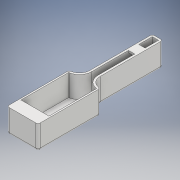
# Autodesk Inventor part: POVwand
Saved by Autodesk Inventor 2017 SP1 (Build 210196100, 196)
## iProperties
Created: 2016-11-21
Part Number: POVwand
Material: ABS Plastic
Document SubType Name: Modeling
Designer: bzs3334
Density: 1.06 g/cm^3
Appearance: Smooth - White
Mass: 17.3028 g
Surface Area: 186.157 cm^2
Volume: 16.3234 cm^3
Author: bzs3334
Autodesk Inventor part; units mm, degrees
ref_plane "YZ Plane" through (0, 0, 0) normal (1, 0, 0) x (0, 1, 0)
ref_plane "XZ Plane" through (0, 0, 0) normal (0, 1, 0) x (-1, 0, 0)
ref_plane "XY Plane" through (0, 0, 0) normal (0, 0, 1) x (1, 0, 0)
sketch "Sketch1" plane through (0, 0, 0) normal (0, 0, 1) x (1, 0, 0)
  line L0 (-5, 0) -> (5, 0)
  line L1 (5, 10) -> (5, 115)
  line L2 (5, 115) -> (-5, 115)
  line L3 (-5, 115) -> (-5, 10)
  line L4 (-15, 0) -> (15, 0)
  line L5 (15, 0) -> (15, -60)
  line L6 (15, -60) -> (-15, -60)
  line L7 (-15, -60) -> (-15, 0)
  arc A0 (-15, 0) -> (-5, 10) centre (-15, 10) ccw
  line L8 (-15, 0) -> (-5, 10) construction
  line L9 (-15, 0) -> (-0.8579, 0) construction
  line L10 (0, 0) -> (0, 115)
  arc A1 (5, 10) -> (15, 0) centre (15, 10) ccw
  circle A2 centre (0, 65) radius 2.7
  circle A3 centre (0, 58.6) radius 2.7
  circle A4 centre (0, 52.2) radius 2.7
  circle A5 centre (0, 45.8) radius 2.7
  circle A6 centre (0, 39.4) radius 2.7
  circle A7 centre (0, 33) radius 2.7
  circle A8 centre (0, 26.6) radius 2.7
  circle A9 centre (0, 20.2) radius 2.7
  circle A10 centre (0, 13.8) radius 2.7
  circle A11 centre (0, 7.4) radius 2.7
  circle A12 centre (0, 1) radius 2.7
  line L11 (5, 68.5) -> (-5, 68.5)
  dimension "a" = 10
  dimension "d1" = 115
  dimension "d2" = 5
  dimension "d3" = 60
  dimension "b" = 30
  dimension "d6" = 15
  dimension "d7" = 45
  dimension "d10" = 5.4
  dimension "d11" = 50
  dimension "d14" = 6.4
  dimension "d47" = 3.5
  constraints: 24 end point, 13 centre point, 4 parallel, 4 point on circle, 4 point on line, 3 horizontal, 3 perpendicular, 2 symmetric about line, 2 tangent, 1 equal length, 1 midpoint, 1 vertical, 21 other
  measures "a" distance between parallel lines of L3 L1
  measures "d1" distance of L0.end L1.end
  measures "d2" distance from line of L10.start L1
  measures "d3" distance of L4.end L5.end
  measures "b" distance of L5.end L6.end
  measures "d6" distance from line of L10.start L5
  measures "d7" angle of L9 L8
  measures "d10" diameter of A2
  measures "d11" distance of L10.end A2.centre
  measures "d14" distance of A2.centre A3.centre
  measures "d47" distance from line of L11 A2.centre
extrude "Extrusion1" add sketch "Sketch1" along normal blind 23
sketch "Sketch2" plane through (0, 0, 23) normal (0, 0, 1) x (1, 0, 0)
  line L0 (5, 115) -> (-5, 115) projected
  line L1 (-5, 115) -> (-5, 10) projected
  arc A0 (-15, 0) -> (-5, 10) centre (-15, 10) ccw projected
  line L2 (-15, 0) -> (-15, -60) projected
  line L3 (-15, -60) -> (15, -60) projected
  line L4 (15, -60) -> (15, 0) projected
  arc A1 (5, 10) -> (15, 0) centre (15, 10) ccw projected
  line L5 (5, 10) -> (5, 115) projected
  line L6 (-13, -28) -> (-13, -1.8322)
  arc A2 (-13, -1.8322) -> (-3, 10) centre (-15, 10) ccw
  line L7 (-3, 10) -> (-3, 113)
  line L8 (-3, 113) -> (3, 113)
  line L9 (3, 113) -> (3, 10)
  arc A3 (3, 10) -> (13, -1.8322) centre (15, 10) ccw
  line L10 (13, -1.8322) -> (13, -28)
  line L11 (-15, 0) -> (-15, -60) projected
  line L12 (-15, -28) -> (13, -28)
  point P0 (0, 0)
  dimension "d19" = 2
  constraints: 12 end point, 4 point on circle, 2 centre point, 1 point on line, 4 other
  measures "d19" distance between parallel lines of L2 L6
extrude "Extrusion2" cut sketch "Sketch2" against normal blind 21 contours L6 A2 L7 L8 L9 A3 L10 L12
sketch "Sketch3" plane through (-13, -28, 23) normal (0, 1, 0) x (1, 0, 0)
  line L0 (-2, 23) -> (28, 23) projected
  line L1 (28, 23) -> (28, 0) projected
  line L2 (-2, 0) -> (28, 0) projected
  line L3 (-2, 23) -> (-2, 0) projected
  line L4 (26, 2) -> (26, 21)
  line L5 (26, 21) -> (0, 21)
  line L6 (0, 21) -> (0, 2)
  line L7 (0, 2) -> (26, 2)
  point P0 (13, 23)
  dimension "d23" = 2
  constraints: 8 end point, 3 other
  measures "d23" distance between parallel lines of L2 L7
extrude "Extrusion3" cut sketch "Sketch3" against normal blind 30 contours L7 L6 L5 L4
extrude "Extrusion4" cut sketch "Sketch1" along normal through all contours A12 L10 L0 | L0 A12 | L10 A12 L0 | A11 L10 | L10 A11 | A10 L10 | L10 A10 | A2 L10 | L10 A2 | A9 L10 | L10 A9 | A3 L10 | L10 A3 | A8 L10 | L10 A8 | A4 L10 | L10 A4 | A7 L10 | L10 A7 | A5 L10 | L10 A5 | A6 L10 | L10 A6
fillet "Fillet1" radius 2 1 edges at (15, 0, 11.5)
mirror "Mirror1" about plane through (0, 0, 0) normal (1, 0, 0) of "Fillet1"
fillet "Fillet2" radius 2 2 edges at (-15, -60, 11.5) (15, -60, 11.5)
fillet "Fillet4" radius 2 2 edges at (5, 115, 11.5) (-5, 115, 11.5)
fillet "Fillet5" radius 2 14 edges at (-7.3624, 3.545, 0) (-14.5275, -0.5412, 0) (-15, -29.9161, 0) (-14.4142, -59.4142, 0) (0, -60, 0) (14.4142, -59.4142, 0) (15, -29.9161, 0) (14.5275, -0.5412, 0) (7.3624, 3.545, 0) (5, 61.5, 0) (4.4142, 114.4142, 0) (0, 115, 0) (-4.4142, 114.4142, 0) (-5, 61.5, 0)
sketch "Sketch4" plane through (-13, -28, 23) normal (1, 0, 0) x (0, 0, -1)
  line L0 (21, -30) -> (21, 26.1678) projected
  line L1 (0, -30) -> (21, -30) projected
  line L2 (0, 26.1678) -> (0, -30) projected
  line L3 (21, 26.1678) -> (0, 26.1678) projected
  point P0 (23, 28)
sketch "Sketch5" plane through (-13, -28, 23) normal (1, 0, 0) x (0, 0, -1)
  line L0 (0, 0) -> (2, 0) projected
  line L1 (2, 0) -> (2, -30) projected
  point P0 (23, 28)
sketch "Sketch6" plane through (-13, -28, 23) normal (0, 1, 0) x (1, 0, 0)
  line L0 (26, 2) -> (0, 2) projected
  line L1 (0, 0) -> (26, 0) projected
  line L2 (26, 0) -> (26, 21) projected
  line L3 (0, 0) -> (26, 0)
  line L4 (26, 0) -> (26, 2)
  line L5 (26, 2) -> (0, 2)
  line L6 (0, 2) -> (0, 0)
  point P0 (13, 23)
  constraints: 8 end point, 2 parallel, 1 horizontal, 1 perpendicular
extrude "Extrusion5" cut sketch "Sketch6" against normal blind 10
extrude "Extrusion6" cut sketch "Sketch4" against normal blind 0.5
mirror "Mirror2" about plane through (0, 0, 0) normal (1, 0, 0) of "Extrusion6"
sketch "Sketch9" plane through (13, -58, 23) normal (1, 0, 0) x (0, 0, -1)
  line L0 (2, 20) -> (2, 0) projected
  line L1 (2, 0) -> (0, 0) projected
  line L2 (0, 20) -> (0, 0) projected
  line L3 (0, 20) -> (2, 20) projected
  point P0 (23, 58)
extrude "Extrusion7" add sketch "Sketch9" along normal blind 0.5
mirror "Mirror3" about plane through (0, 0, 0) normal (1, 0, 0) of "Extrusion7"
sketch "Sketch10" plane through (0, 0, 23) normal (0, 0, 1) x (1, 0, 0)
  arc A0 (-3, 115) -> (-5, 113) centre (-3, 113) ccw projected
  line L0 (-5, 113) -> (-5, 10) projected
  arc A1 (-13.3333, 0.1399) -> (-5, 10) centre (-15, 10) ccw projected
  arc A2 (-13.3333, 0.1399) -> (-15, -1.8322) centre (-13, -1.8322) ccw projected
  line L1 (-15, -1.8322) -> (-15, -58) projected
  arc A3 (-15, -58) -> (-13, -60) centre (-13, -58) ccw projected
  line L2 (-13, -60) -> (13, -60) projected
  arc A4 (13, -60) -> (15, -58) centre (13, -58) ccw projected
  line L3 (15, -58) -> (15, -1.8322) projected
  arc A5 (15, -1.8322) -> (13.3333, 0.1399) centre (13, -1.8322) ccw projected
  arc A6 (5, 10) -> (13.3333, 0.1399) centre (15, 10) ccw projected
  line L4 (5, 10) -> (5, 113) projected
  arc A7 (5, 113) -> (3, 115) centre (3, 113) ccw projected
  line L5 (3, 115) -> (-3, 115) projected
  line L6 (13, -1.8322) -> (13.5, -1.8322) projected
  line L7 (13.5, -1.8322) -> (13.5, -38) projected
  line L8 (13.5, -38) -> (-13.5, -38) projected
  line L9 (-13.5, -38) -> (-13.5, -1.8322) projected
  line L10 (-13.5, -1.8322) -> (-13, -1.8322) projected
  arc A8 (-13, -1.8322) -> (-3, 10) centre (-15, 10) ccw projected
  line L11 (-3, 10) -> (-3, 113) projected
  line L12 (-3, 113) -> (3, 113) projected
  line L13 (3, 113) -> (3, 10) projected
  arc A9 (3, 10) -> (13, -1.8322) centre (15, 10) ccw projected
  line L14 (-13.5, -38) -> (-13.5, -1.8322) projected
  line L15 (13.5, -58) -> (13.5, -38) projected
  line L16 (-13.5, -38) -> (13.5, -38)
  line L17 (13.5, -38) -> (13.5, -48)
  line L18 (13.5, -48) -> (-13.5, -48)
  line L19 (-13.5, -48) -> (-13.5, -38)
  point P0 (0, 0)
  dimension "d53" = 10
  constraints: 8 end point, 2 parallel, 1 horizontal, 1 midpoint, 1 perpendicular
  measures "d53" distance of L16.end L17.end
sketch "Sketch11" plane through (-13, -38, 23) normal (0, 1, 0) x (1, 0, 0)
  line L0 (-0.5, 2) -> (26.5, 2) projected
  line L1 (26, 21) -> (0, 21) projected
  line L2 (26, 0) -> (26, 21) projected
  line L3 (0, 0) -> (26, 0) projected
  line L4 (0, 21) -> (0, 0) projected
  line L5 (0, 21) -> (0, 0) projected
  line L6 (26, 0) -> (26, 21) projected
  line L7 (0, 2) -> (26, 2)
  line L8 (26, 2) -> (26, 1.5)
  line L9 (26, 1.5) -> (0, 1.5)
  line L10 (0, 1.5) -> (0, 2)
  line L11 (-0.5, 21) -> (-0.5, 2) projected
  line L12 (0, 1.5) -> (-0.5, 1.5)
  line L13 (-0.5, 1.5) -> (-0.5, 2)
  line L14 (-0.5, 2) -> (0, 2)
  line L15 (0, 2) -> (0, 1.5)
  point P0 (13, 23)
  dimension "d39" = 0.5
  constraints: 16 end point, 4 parallel, 3 point on line, 2 horizontal, 2 perpendicular
  measures "d39" distance of L7.end L8.end
extrude "Extrusion8" cut sketch "Sketch11" against normal blind 20 contours L0 L4 L12 L13 | L0 L2 L9 L4
sketch "Sketch12" plane through (-3, 10, 23) normal (1, 0, 0) x (0, 0, -1)
  line L0 (21, 0) -> (21, 103) projected
  line L1 (21, 0) -> (0, 0) projected
  line L2 (0, 103) -> (0, 0) projected
  line L3 (21, 103) -> (0, 103) projected
  line L4 (0, 103) -> (0, 0) projected
  line L5 (0, 35.5) -> (2, 35.5)
  line L6 (2, 35.5) -> (2, 45.5)
  line L7 (2, 45.5) -> (0, 45.5)
  line L8 (0, 45.5) -> (0, 35.5)
  point P0 (23, -10)
  dimension "d42" = 2
  dimension "d43" = 10
  dimension "d44" = 57.5
  constraints: 8 end point, 2 parallel, 1 horizontal, 1 perpendicular, 1 point on line
  measures "d42" distance of L7.end L6.end
  measures "d43" distance of L6.end L5.end
  measures "d44" distance between parallel lines of L3 L7
extrude "Extrusion9" add sketch "Sketch12" along normal through all contours L2 L7 L6 L5
extrude "Extrusion10" cut sketch "Sketch1" along normal through all contours L3 L2 L10 L11 | L10 L2 L1 L11
sketch "Sketch13" plane through (-3, 68.5, 0) normal (0, 1, 0) x (1, 0, 0)
  line L0 (8, -23) -> (6, -23) projected
  line L1 (8, -2) -> (8, -23) projected
  arc A0 (8, -2) -> (6, 0) centre (6, -2) ccw projected
  line L2 (0, 0) -> (6, 0) projected
  arc A1 (0, 0) -> (-2, -2) centre (0, -2) ccw projected
  line L3 (-2, -23) -> (-2, -2) projected
  line L4 (0, -23) -> (-2, -23) projected
  line L5 (0, -2) -> (0, -23) projected
  line L6 (6, -2) -> (0, -2) projected
  line L7 (6, -23) -> (6, -2) projected
  line L8 (-10, -23) -> (0, -23) projected
  line L9 (6, -2) -> (0, -2)
  line L10 (0, -2) -> (0, -23)
  line L11 (0, -23) -> (6, -23)
  line L12 (6, -23) -> (6, -2)
  point P0 (3, 0)
  constraints: 8 end point, 2 parallel, 1 horizontal, 1 perpendicular
extrude "Extrusion11" add sketch "Sketch13" along normal blind 2
fillet "Fillet6" radius 2 5 edges at (4.4142, 70.5, 0.5858) (0, 70.5, 0) (-4.4142, 70.5, 0.5858) (-5, 70.5, 12.5) (5, 70.5, 12.5)
extrude "Extrusion12" cut sketch "Sketch10" against normal blind 2 contours L15 L18 L19 L8
equation "\"d2\" = 0.5 * a"
equation "\"d6\" = 0.5 * b"
body "Solid1"
